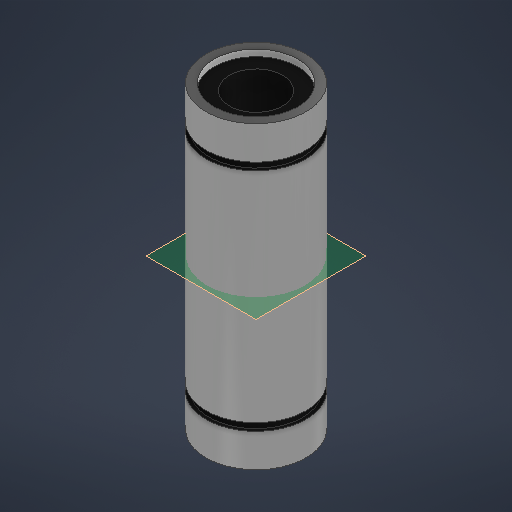
# Autodesk Inventor part: Linear Bearing 8mm Round
Saved by Autodesk Inventor 2025.1 (Build 291241000, 241)
## iProperties
Created: 2024-11-10
Part Number: Linear Bearing 8mm Round
Material: Generic
Document SubType Name: Modeling
Designer: jerem
Density: 1 g/cm^3
Appearance: Default
Author: jerem
Autodesk Inventor part; units mm, degrees
ref_plane "YZ Plane" through (0, 0, 0) normal (1, 0, 0) x (0, 1, 0)
ref_plane "XZ Plane" through (0, 0, 0) normal (0, 1, 0) x (-1, 0, 0)
ref_plane "XY Plane" through (0, 0, 0) normal (0, 0, 1) x (1, 0, 0)
sketch "Sketch1" plane through (0, 0, 0) normal (0, 1, 0) x (-1, 0, 0)
  circle A0 centre (0, 0) radius 4
  circle A1 centre (0, 0) radius 7.5
  circle A2 centre (0, 0) radius 6.25
  circle A3 centre (0, 0) radius 7
  dimension "d0" = 8
  dimension "d1" = 15
  dimension "d2" = 12.5
  dimension "d13" = 0.5
  constraints: 4 centre point, 4 coincident
  measures "d0" diameter of A0
  measures "d1" diameter of A1
  measures "d2" diameter of A2
  measures "d13" radial gap between concentric circles of A3 A1
extrude "Extrusion1" add sketch "Sketch1" along normal blind 45 contours A2 | A3
ref_plane "Work Plane1" through (0, 22.5, 0) normal (0, -1, 0) x (1, 0, 0)
extrude "Extrusion2" add sketch "Sketch1" along normal mid plane 32.75 from surface at 22.5 contours A1
extrude "Extrusion3" add sketch "Sketch1" along normal blind 5 contours A1
extrude "Extrusion5" cut sketch "Sketch1" along normal blind 1 contours A2
mirror "Mirror1" about plane through (0, 22.5, 0) normal (0, -1, 0) of "Extrusion3", "Extrusion5"
body "Solid1"
